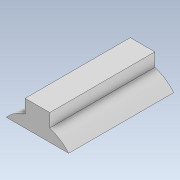
# Autodesk Inventor part: Flansch_Flachstelle
Saved by Autodesk Inventor 2022 (Build 260153000, 153)
## iProperties
Created: 2022-09-13
Part Number: Flansch_Flachstelle
Material: Generisch
Document SubType Name: Modeling
Designer: alexw
Density: 1 g/cm^3
Appearance: Vorgabe
D: 20,000 mm
Wellennuttiefe_20: 3,500 mm
Nabennuttiefe_20: 2,800 mm
Passfeder_Width_20: 6,000 mm
Author: alexw
Autodesk Inventor part; units mm, degrees
note: some values were not read from the file. Left out: dimensions or parameters whose unit could not be read.
ref_plane "YZ Plane" through (0, 0, 0) normal (1, 0, 0) x (0, 1, 0)
ref_plane "XZ Plane" through (0, 0, 0) normal (0, 1, 0) x (-1, 0, 0)
ref_plane "XY Plane" through (0, 0, 0) normal (0, 0, 1) x (1, 0, 0)
sketch "Skizze1" plane through (0, 0, 0) normal (0, 0, 1) x (1, 0, 0)
  line L0 (0, 0) -> (0, 6.3) construction
  line L1 (-3, 6.3) -> (3, 6.3)
  circle A0 centre (0, -6.5) radius 10 construction
  line L2 (3, 6.3) -> (3, 3.0394)
  line L3 (7.5993, 0) -> (-7.5993, 0)
  line L4 (-3, 6.3) -> (-3, 3.0394)
  line L5 (-3, 3.0394) -> (3, 3.0394) construction
  arc A1 (-3, 3.0394) -> (-7.5993, 0) centre (0, -6.5) ccw
  arc A2 (7.5993, 0) -> (3, 3.0394) centre (0, -6.5) ccw
  point P0 (0, 3.5)
  dimension "d0" = 20
  dimension "d1" = 2.8
  dimension "d2" = 3.5
  dimension "d3" = 6
  constraints: 12 end point, 7 point on circle, 3 centre point, 3 vertical, 2 concentric, 2 horizontal, 2 midpoint, 2 point on line, 1 perpendicular
  measures "d0" diameter of A0
  measures "d1" distance from line of L1 point (0, 3.5)
  measures "d2" distance from line of L3 point (0, 3.5)
  measures "d3" distance between parallel lines of L2 L4
extrude "Extrusion1" add sketch "Skizze1" along normal blind 25.6
equation "\"d0\" = D"
equation "\"d1\" = Nabennuttiefe_20"
equation "\"d2\" = Wellennuttiefe_20"
equation "\"d3\" = Passfeder_Width_20"
equation "\"Passfeder_Width_20\" = 6"
equation "\"Nabennuttiefe_20\" = 2.8"
equation "\"Wellennuttiefe_20\" = 3.5"
